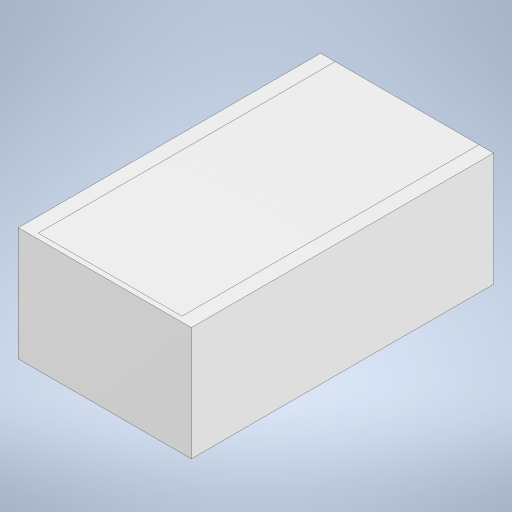
# Autodesk Inventor part: razerbasilisku
Saved by Autodesk Inventor 2024.1 (Build 281209000, 209)
## iProperties
Created: 2023-12-29
Part Number: razerbasilisku
Material: ABS Plastic
Document SubType Name: Modeling
Designer: tomma
Density: 1.06 g/cm^3
Appearance: Smooth - White
Author: tomma
Autodesk Inventor part; units mm, degrees
ref_plane "YZ Plane" through (0, 0, 0) normal (1, 0, 0) x (0, 1, 0)
ref_plane "XZ Plane" through (0, 0, 0) normal (0, 1, 0) x (-1, 0, 0)
ref_plane "XY Plane" through (0, 0, 0) normal (0, 0, 1) x (1, 0, 0)
sketch "Sketch2" plane through (0, 0, 0) normal (0, 0, 1) x (1, 0, 0)
  line L0 (-39.0745, 47.4918) -> (38.9255, 47.4918) construction
  line L1 (38.9255, 47.4918) -> (38.9255, 37.6976) construction
  line L2 (38.9255, 2.4918) -> (-39.0745, 2.4918)
  line L3 (-39.0745, 2.4918) -> (-39.0745, 37.6976)
  line L4 (-41.5745, 54.4918) -> (-34.5745, 54.4918)
  line L5 (41.4255, 54.4918) -> (41.4255, -0.0082)
  line L6 (41.4255, -0.0082) -> (-41.5745, -0.0082)
  line L7 (-41.5745, -0.0082) -> (-41.5745, 54.4918)
  line L8 (-0.0745, 2.4918) -> (-0.0745, -0.0082)
  line L9 (-34.5745, 54.4918) -> (-34.5745, 52.4918)
  line L10 (-34.5745, 54.4918) -> (-34.5745, 52.4918)
  line L11 (-34.5745, 52.4918) -> (-35.5745, 52.4918)
  line L12 (-39.5745, 48.4918) -> (-39.5745, 47.4918)
  line L13 (-39.5745, 47.4918) -> (-34.5745, 47.4918)
  line L14 (-39.5745, 48.4918) -> (-35.5745, 52.4918)
  line L15 (34.4255, 54.4918) -> (34.4255, 52.4918)
  line L16 (34.4255, 54.4918) -> (34.4255, 52.4918)
  line L17 (34.4255, 52.4918) -> (35.4255, 52.4918)
  line L18 (39.4255, 48.4918) -> (39.4255, 47.4918)
  line L19 (39.4255, 47.4918) -> (34.4255, 47.4918)
  line L20 (39.4255, 48.4918) -> (35.4255, 52.4918)
  line L21 (-34.5745, 47.4918) -> (-34.5745, 45.4918)
  line L22 (-34.5745, 45.4918) -> (-39.0745, 37.6976)
  line L23 (-34.5745, 45.4918) -> (-24.5745, 45.4918) construction
  line L24 (-34.5745, 52.4918) -> (-34.5745, 47.4918) construction
  line L25 (-34.5745, 54.4918) -> (34.4255, 54.4918) construction
  line L26 (34.4255, 54.4918) -> (41.4255, 54.4918)
  line L27 (34.4255, 47.4918) -> (34.4255, 45.4918)
  line L28 (34.4255, 45.4918) -> (38.9255, 37.6976)
  line L29 (34.4255, 54.4918) -> (-34.5745, 54.4918) construction
  line L30 (34.4255, 52.4918) -> (34.4255, 47.4918) construction
  line L31 (-39.0745, 37.6976) -> (-39.0745, 47.4918) construction
  line L32 (38.9255, 37.6976) -> (38.9255, 2.4918)
  point P0 (-39.5745, 52.4918)
  dimension "d13" = 78
  dimension "d14" = 45
  dimension "d15" = 83
  dimension "d16" = 54.5
  dimension "d17" = 2.5
  dimension "d18" = 7
  dimension "d19" = 7
  dimension "d20" = 2
  dimension "d21" = 5
  dimension "d22" = 5
  dimension "d23" = 5
  dimension "d24" = 4
  dimension "d25" = 4
  dimension "d26" = 2
  dimension "d28" = 120
  constraints: 66 end point, 10 symmetric about line, 9 parallel, 8 perpendicular, 5 horizontal, 3 vertical, 2 midpoint, 2 point on line
  measures "d13" distance of L2.start L2.end
  measures "d14" distance of L0.end L2.start
  measures "d15" distance of L5.end L6.end
  measures "d16" distance of L5.start L5.end
  measures "d17" distance of L8.end L8.start
  measures "d18" distance of L4.end L13.end
  measures "d19" distance between parallel lines of L7 L9
  measures "d20" distance of L4.end L9.end
  measures "d21" distance of L9.end point (-39.575, 52.492)
  measures "d22" distance of point (-39.575, 52.492) L12.end
  measures "d23" distance of L12.end L13.end
  measures "d24" distance of L12.start point (-39.575, 52.492)
  measures "d25" distance of L11.end point (-39.575, 52.492)
  measures "d26" distance of L13.end L21.end
  measures "d28" angle of L22 L23
extrude "Extrusion1" add sketch "Sketch2" along normal mid plane 140
sketch "Sketch3" plane through (0, 0, 70) normal (0, 0, 1) x (1, 0, 0)
  line L0 (-34.5745, 54.4918) -> (-41.5745, 54.4918) projected
  line L1 (41.4255, -0.0082) -> (41.4255, 54.4918) projected
  line L2 (-41.5745, 54.4918) -> (41.4255, 54.4918)
  line L3 (41.4255, 54.4918) -> (41.4255, -0.0082)
  line L4 (41.4255, -0.0082) -> (-41.5745, -0.0082)
  line L5 (-41.5745, -0.0082) -> (-41.5745, 54.4918)
  point P0 (0, 0)
  constraints: 8 end point, 2 parallel, 1 horizontal, 1 perpendicular
extrude "Extrusion2" add sketch "Sketch3" along normal blind 2.5
sketch "Sketch4" plane through (0, 0, -70) normal (0, 0, -1) x (-1, 0, 0)
  line L0 (34.5745, 45.4918) -> (39.0745, 37.6976) projected
  line L1 (39.0745, 37.6976) -> (39.0745, 2.4918) projected
  line L2 (39.0745, 2.4918) -> (-38.9255, 2.4918) projected
  line L3 (-38.9255, 2.4918) -> (-38.9255, 37.6976) projected
  line L4 (-38.9255, 37.6976) -> (-34.4255, 45.4918) projected
  line L5 (-34.4255, 45.4918) -> (-34.4255, 47.4918) projected
  line L6 (-34.4255, 47.4918) -> (-39.4255, 47.4918) projected
  line L7 (-39.4255, 47.4918) -> (-39.4255, 48.4918) projected
  line L8 (-39.4255, 48.4918) -> (-35.4255, 52.4918) projected
  line L9 (-35.4255, 52.4918) -> (-34.4255, 52.4918) projected
  line L10 (-34.4255, 52.4918) -> (-34.4255, 54.4918) projected
  line L11 (-34.4255, 54.4918) -> (-41.4255, 54.4918) projected
  line L12 (-41.4255, 54.4918) -> (-41.4255, -0.0082) projected
  line L13 (-41.4255, -0.0082) -> (41.5745, -0.0082) projected
  line L14 (41.5745, -0.0082) -> (41.5745, 54.4918) projected
  line L15 (41.5745, 54.4918) -> (34.5745, 54.4918) projected
  line L16 (34.5745, 54.4918) -> (34.5745, 52.4918) projected
  line L17 (34.5745, 52.4918) -> (35.5745, 52.4918) projected
  line L18 (35.5745, 52.4918) -> (39.5745, 48.4918) projected
  line L19 (39.5745, 48.4918) -> (39.5745, 47.4918) projected
  line L20 (39.5745, 47.4918) -> (34.5745, 47.4918) projected
  line L21 (34.5745, 47.4918) -> (34.5745, 45.4918) projected
  line L22 (-38.9255, 37.6976) -> (-38.9255, 47.4918)
  line L23 (39.0745, 37.6976) -> (39.0745, 47.4918)
  line L24 (39.0745, 47.4918) -> (-38.9255, 47.4918)
  constraints: 6 end point, 3 perpendicular, 2 point on line
extrude "Extrusion3" add sketch "Sketch4" along normal blind 2.5
sketch "Sketch7" plane through (0, 0, -72.5) normal (0, 0, -1) x (-1, 0, 0)
  line L0 (-39.4255, 47.4918) -> (-39.4255, 48.4918) projected
  line L1 (-39.4255, 48.4918) -> (-35.4255, 52.4918) projected
  line L2 (-35.4255, 52.4918) -> (-34.4255, 52.4918) projected
  line L3 (-34.4255, 52.4918) -> (-34.4255, 54.4918) projected
  line L4 (-34.4255, 54.4918) -> (-41.4255, 54.4918) projected
  line L5 (-41.4255, 54.4918) -> (-41.4255, -0.0082) projected
  line L6 (-41.4255, -0.0082) -> (41.5745, -0.0082) projected
  line L7 (41.5745, -0.0082) -> (41.5745, 54.4918) projected
  line L8 (41.5745, 54.4918) -> (34.5745, 54.4918) projected
  line L9 (34.5745, 54.4918) -> (34.5745, 52.4918) projected
  line L10 (34.5745, 52.4918) -> (35.5745, 52.4918) projected
  line L11 (35.5745, 52.4918) -> (39.5745, 48.4918) projected
  line L12 (39.5745, 48.4918) -> (39.5745, 47.4918) projected
  line L13 (39.5745, 47.4918) -> (-39.4255, 47.4918) projected
  line L14 (-34.4255, 54.4918) -> (34.5745, 54.4918)
  line L15 (-39.4255, 47.4918) -> (-39.4255, 47.9918)
  line L16 (-39.4255, 47.9918) -> (39.5745, 47.9918)
  point P0 (0, 0)
  constraints: 6 end point, 2 midpoint, 1 collinear
extrude "Extrusion5" add sketch "Sketch7" against normal up to next separate body contours L0 L1 L2 L3 L14 L9 L10 L11 L12 L16
equation "\"d25\" = d24"
body "Solid1"
